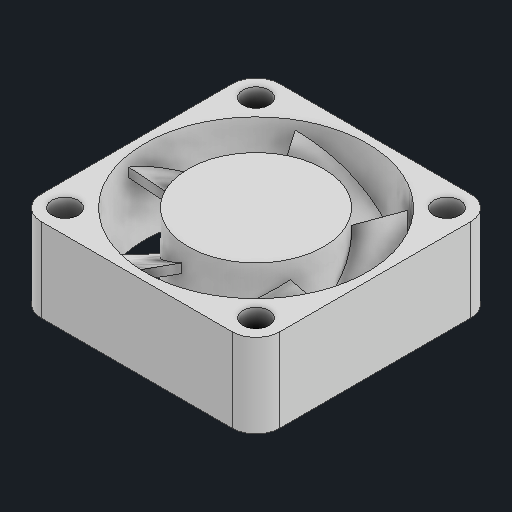
# Autodesk Inventor part: 팬
Saved by Autodesk Inventor 2027.1 (Build 311270010, 270A)
## iProperties
Created: 2026-08-07
Part Number: 팬
Material: 일반
Document SubType Name: Modeling
Designer: moieboy9999
Density: 1.711 g/cm^3
Appearance: 기본값
Mass: 9 g
Surface Area: 48.1735 cm^2
Volume: 5.26008 cm^3
Author: moieboy9999
Autodesk Inventor part; units mm, degrees
ref_plane "YZ Plane" through (0, 0, 0) normal (1, 0, 0) x (0, 1, 0)
ref_plane "XZ Plane" through (0, 0, 0) normal (0, 1, 0) x (-1, 0, 0)
ref_plane "XY Plane" through (0, 0, 0) normal (0, 0, 1) x (1, 0, 0)
sketch "스케치1" plane through (0, 0, 0) normal (0, 1, 0) x (-1, 0, 0)
  line L0 (0, 0) -> (-30, 0)
  line L1 (-30, 0) -> (-30, -30)
  line L2 (-30, -30) -> (0, -30)
  line L3 (0, -30) -> (0, 0)
  line L4 (0, 0) -> (-3, 0)
  line L5 (-3, 0) -> (-3, -3)
  line L6 (-3, -3) -> (0, -3)
  line L7 (0, -3) -> (0, 0)
  circle A0 centre (-3, -3) radius 1.65
  circle A1 centre (-3, -27) radius 1.65
  circle A2 centre (-27, -3) radius 1.65
  circle A3 centre (-27, -27) radius 1.65
  circle A4 centre (-15, -15) radius 14
  dimension "d0" = 30
  dimension "d1" = 30
  dimension "d2" = 3
  dimension "d3" = 3
  dimension "d4" = 3.3
  dimension "d7" = 24
  dimension "d10" = 24
  dimension "d13" = 28
  constraints: 16 end point, 5 centre point, 4 parallel, 3 horizontal, 2 perpendicular, 1 coincident, 1 vertical, 6 other
  measures "d0" distance of L2.end L1.end
  measures "d1" distance of L1.end L0.end
  measures "d2" distance of L6.end L5.end
  measures "d3" distance of L5.end L4.end
  measures "d4" diameter of A0
  measures "d7" distance of A0.centre A1.centre
  measures "d10" distance of A0.centre A2.centre
  measures "d13" diameter of A4
extrude "돌출1" add sketch "스케치1" along normal blind 10.5 contours L3 L6 A0 L5 L0 | L5 A0 L6 L3 L2 L1 L0
fillet "모깎기1" radius 3 4 edges at (30, 5.25, 0) (30, 5.25, -30) (0, 5.25, -30) (0, 5.25, 0)
sketch "스케치2" plane through (0, 10.5, 0) normal (0, 1, 0) x (1, 0, 0)
  circle A0 centre (15, 15) radius 14 projected
  circle A1 centre (15, 15) radius 8.5
  line L0 (15, 15) -> (14.5, 15)
  line L1 (14.5, 15) -> (15.5, 15)
  line L2 (15.5, 15) -> (15.5, 28.5)
  line L3 (15.5, 28.5) -> (14.5, 28.5)
  line L4 (14.5, 28.5) -> (14.5, 15)
  point P0 (0, 0)
  dimension "d17" = 17
  dimension "d18" = 0.5
  dimension "d19" = 1
  dimension "d20" = 13.5
  constraints: 10 end point, 2 horizontal, 2 parallel, 1 centre point, 1 coincident, 1 perpendicular
  measures "d17" diameter of A1
  measures "d18" distance of L0.start L0.end
  measures "d19" distance of L3.end L2.end
  measures "d20" distance of L2.end L1.end
extrude "돌출2" add sketch "스케치2" against normal blind 10.5 contours A1 L4 L0 L1 L2 | L2 L1 L0 L4 A1
extrude "돌출3" add sketch "스케치2" against normal blind 10.5 separate body contours L2 L1 L0 L4 A1 | A1 L4 L3 L2 picked at (15.3333, 17.8284)
move faces "회전1" rotation origin (0, 0, 0) rotation axis (0, 0, 1) rotation angle 60 translate (12.0466, -10.3654, 0) faces at (15.1667, 7, -28.5) (14.5, 7, -24) (15.5, 7, -19.5)
sketch "스케치3" plane through (15, 0, -15) normal (0, -1, 0) x (1, 0, 0)
  circle A0 centre (0, 0) radius 8.5 projected
  circle A1 centre (0, 0) radius 8.5
  line L0 (0, 0) -> (15, -25.9808)
  line L1 (0, 0) -> (30, 0) construction
  line L2 (0, 0) -> (-15, -25.9808)
  line L3 (0, 0) -> (30, 0) construction
  line L4 (-15, -25.9808) -> (15, -25.9808)
  circle A2 centre (0, 0) radius 13.5
  line L5 (-10.0933, -13.5) -> (8.0933, -13.5) projected
  point P0 (-15, 15)
  point P1 (4.25, -7.3612)
  point P2 (-4.25, -7.3612)
  point P3 (-6.75, -11.6913)
  point P4 (6.75, -11.6913)
  dimension "d26" = 30
  dimension "d27" = 60
  dimension "d28" = 120
  constraints: 10 end point, 3 horizontal, 2 centre point, 2 coincident, 2 equal length, 1 tangent
  measures "d26" distance of L0.start L0.end
  measures "d27" angle of L0 L1
  measures "d28" angle of L2 L3
extrude "돌출4" add sketch "스케치3" against normal blind 10.5 separate body contours A0 L0 A2 L2 picked at (5.2058, -10.5795)
combine bodies "결합1" operation type common bodies to combine 2 3
pattern_circular "원형 패턴1" count 5 over 360 about axis through (15, 10.5, -15) along (0, -1, 0) bodies 2
combine bodies "결합2" operation type add bodies to combine 1 2
